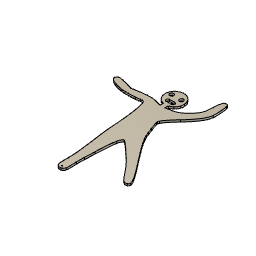
human (Autodesk Fusion 360 design; units mm, degrees)
Autodesk Fusion 360 part; units mm, degrees
sketch "Sketch1" plane through (0, 0, 0) normal (0, 1, 0) x (1, 0, 0)
  spline S0 degree 3 poles (28.5505, 138.7144) (26.7377, 138.2108) (26.0126, 135.8139) (25.6097, 128.7641) knots 0 0 0 0 1 1 1 1
  spline S1 degree 3 poles (25.6097, 128.7641) (25.1062, 119.7605) (24.5019, 117.988) (20.3324, 113.3552) knots 0 0 0 0 1 1 1 1
  spline S2 degree 3 poles (20.3324, 113.3552) (14.6322, 107.0104) (12.2151, 105.7213) (3.1309, 104.1703) knots 0 0 0 0 1 1 1 1
  spline S3 degree 3 poles (3.1309, 104.1703) (-1.1191, 103.4654) (-3.1132, 103.4654) (-5.5101, 104.1905) knots 0 0 0 0 1 1 1 1
  spline S4 degree 3 poles (-5.5101, 104.1905) (-13.4462, 106.6277) (-16.2057, 106.668) (-28.8752, 104.5732) knots 0 0 0 0 1 1 1 1
  line L0 (-28.8752, 104.5732) -> (-33.3267, 103.8481)
  line L1 (-33.3267, 103.8481) -> (-36.8314, 104.8552)
  spline S5 degree 3 poles (-36.8314, 104.8552) (-44.1632, 106.9701) (-47.4061, 107.6348) (-49.1182, 107.3931) knots 0 0 0 0 1 1 1 1
  spline S6 degree 3 poles (-49.1182, 107.3931) (-50.9915, 107.1111) (-51.918, 105.1775) (-50.931, 103.6064) knots 0 0 0 0 1 1 1 1
  spline S7 degree 3 poles (-50.931, 103.6064) (-49.6218, 101.4713) (-43.5388, 99.0945) (-37.2343, 98.2284) knots 0 0 0 0 1 1 1 1
  spline S8 degree 3 poles (-37.2343, 98.2284) (-34.5956, 97.8658) (-26.9818, 97.9262) (-23.4368, 98.3291) knots 0 0 0 0 1 1 1 1
  spline S9 degree 3 poles (-23.4368, 98.3291) (-21.8858, 98.4902) (-19.6702, 98.7521) (-18.5019, 98.8729) knots 0 0 0 0 1 1 1 1
  spline S10 degree 3 poles (-18.5019, 98.8729) (-15.259, 99.2556) (-15.1986, 99.2153) (-14.1915, 96.1336) knots 0 0 0 0 1 1 1 1
  spline S11 degree 3 poles (-14.1915, 96.1336) (-12.3384, 90.4534) (-10.6464, 78.8917) (-9.74, 65.618) knots 0 0 0 0 1 1 1 1
  spline S12 degree 3 poles (-9.74, 65.618) (-9.1358, 56.8762) (-8.3502, 49.6048) (-7.1215, 41.3465) knots 0 0 0 0 1 1 1 1
  spline S13 degree 3 poles (-7.1215, 41.3465) (-6.5173, 37.318) (-5.7518, 31.4365) (-4.4829, 20.902) knots 0 0 0 0 1 1 1 1
  spline S14 degree 3 poles (-4.4829, 20.902) (-4.2613, 19.049) (-4.1002, 15.5039) (-3.9995, 9.8238) knots 0 0 0 0 1 1 1 1
  spline S15 degree 3 poles (-3.9995, 9.8238) (-3.8383, 0.3972) (-3.7779, -0.1265) (-2.4082, -1.4761) knots 0 0 0 0 1 1 1 1
  spline S16 degree 3 poles (-2.4082, -1.4761) (-1.5018, -2.3825) (-0.2933, -2.6443) (1.3584, -2.2818) knots 0 0 0 0 1 1 1 1
  spline S17 degree 3 poles (1.3584, -2.2818) (2.7079, -1.9796) (3.4935, -1.1336) (3.856, 0.377) knots 0 0 0 0 1 1 1 1
  spline S18 degree 3 poles (3.856, 0.377) (4.1582, 1.5856) (4.1783, 5.2515) (3.9567, 10.7302) knots 0 0 0 0 1 1 1 1
  spline S19 degree 3 poles (3.9567, 10.7302) (3.8762, 12.6638) (3.9165, 16.3096) (4.0373, 19.0087) knots 0 0 0 0 1 1 1 1
  spline S20 degree 3 poles (4.0373, 19.0087) (4.1582, 21.6473) (4.3596, 26.2196) (4.4603, 29.1604) knots 0 0 0 0 1 1 1 1
  spline S21 degree 3 poles (4.4603, 29.1604) (4.8631, 38.9093) (5.4674, 46.2008) (6.1925, 49.6451) knots 0 0 0 0 1 1 1 1
  spline S22 degree 3 poles (6.1925, 49.6451) (6.8371, 52.747) (7.8442, 54.5397) (8.952, 54.5397) knots 0 0 0 0 1 1 1 1
  spline S23 degree 3 poles (8.952, 54.5397) (9.7174, 54.5397) (13.9876, 50.8738) (22.4272, 42.9176) knots 0 0 0 0 1 1 1 1
  spline S24 degree 3 poles (22.4272, 42.9176) (30.464, 35.3441) (34.0494, 31.4365) (39.9108, 23.9234) knots 0 0 0 0 1 1 1 1
  spline S25 degree 3 poles (39.9108, 23.9234) (44.8255, 17.5987) (46.6383, 16.37) (49.1158, 17.639) knots 0 0 0 0 1 1 1 1
  spline S26 degree 3 poles (49.1158, 17.639) (50.1833, 18.203) (50.4653, 18.7065) (50.3042, 19.8345) knots 0 0 0 0 1 1 1 1
  spline S27 degree 3 poles (50.3042, 19.8345) (49.9013, 22.7954) (46.3362, 28.113) (34.7745, 43.0586) knots 0 0 0 0 1 1 1 1
  spline S28 degree 3 poles (34.7745, 43.0586) (22.5682, 58.8099) (18.2981, 65.054) (15.8407, 70.6535) knots 0 0 0 0 1 1 1 1
  spline S29 degree 3 poles (15.8407, 70.6535) (13.8265, 75.2863) (10.6641, 83.8065) (9.9793, 86.4854) knots 0 0 0 0 1 1 1 1
  line L2 (9.9793, 86.4854) -> (9.6167, 87.8954)
  line L3 (9.6167, 87.8954) -> (10.2411, 89.2046)
  spline S30 degree 3 poles (10.2411, 89.2046) (11.349, 91.5411) (14.3905, 95.3883) (19.849, 101.2497) knots 0 0 0 0 1 1 1 1
  spline S31 degree 3 poles (19.849, 101.2497) (28.4699, 110.5555) (31.9143, 116.0543) (32.6797, 121.7546) knots 0 0 0 0 1 1 1 1
  spline S32 degree 3 poles (32.6797, 121.7546) (33.0825, 124.8565) (32.5387, 133.1148) (31.6726, 136.4987) knots 0 0 0 0 1 1 1 1
  spline S33 degree 3 poles (31.6726, 136.4987) (31.451, 137.4051) (31.2093, 137.9087) (30.8467, 138.1706) knots 0 0 0 0 1 1 1 1
  spline S34 degree 3 poles (30.8467, 138.1706) (30.1417, 138.6741) (29.2353, 138.8957) (28.5505, 138.7144) knots 0 0 0 0 1 1 1 1
  spline S35 degree 3 poles (-3.9793, 125.924) (-6.5173, 125.2392) (-9.1156, 123.1645) (-10.2234, 120.9287) knots 0 0 0 0 1 1 1 1
  spline S36 degree 3 poles (-10.2234, 120.9287) (-12.8419, 115.591) (-10.2637, 109.2261) (-4.7246, 107.3125) knots 0 0 0 0 1 1 1 1
  spline S37 degree 3 poles (-4.7246, 107.3125) (-1.2803, 106.1241) (2.3856, 106.9097) (5.0243, 109.4073) knots 0 0 0 0 1 1 1 1
  spline S38 degree 3 poles (5.0243, 109.4073) (6.394, 110.6763) (7.1392, 111.8244) (7.7032, 113.4962) knots 0 0 0 0 1 1 1 1
  spline S39 degree 3 poles (7.7032, 113.4962) (8.0658, 114.5839) (8.1262, 115.1479) (8.0456, 116.9406) knots 0 0 0 0 1 1 1 1
  spline S40 degree 3 poles (8.0456, 116.9406) (7.9852, 118.9347) (7.9248, 119.2166) (7.1997, 120.6669) knots 0 0 0 0 1 1 1 1
  spline S41 degree 3 poles (7.1997, 120.6669) (5.1653, 124.8766) (0.4117, 127.1124) (-3.9793, 125.924) knots 0 0 0 0 1 1 1 1
  line L4 (1.3199, 107.2081) -> (1.3199, 103.8951)
  line L5 (-3.5162, 106.9777) -> (-3.5162, 103.7492)
  circle A0 centre (3, 119) radius 2
  circle A1 centre (-7, 119) radius 2
  line L6 (-4, 110.2788) -> (1.4991, 110.2788)
  arc A2 (1.4991, 110.2788) -> (1.4991, 113.7212) centre (1.4991, 112) ccw
  line L7 (1.4991, 113.7212) -> (-4, 113.7212)
  arc A3 (-4, 113.7212) -> (-4, 110.2788) centre (-4, 112) ccw
  line L8 (-4, 112) -> (1.4991, 112) construction
  dimension "d1" = 4
  dimension "d2" = 4
  constraint coincident S37 L4.start
  constraint coincident S3 L4.end
  constraint vertical L4
  constraint coincident S37 L5.start
  constraint coincident S3 L5.end
  constraint parallel L4 L5
  constraint tangent L6 A2
  constraint tangent A2 L7
  constraint parallel L6 L7
  constraint tangent L7 A3
  constraint tangent L6 A3
  constraint horizontal L8
  measures "d1" diameter of A0
  measures "d2" diameter of A1
extrude "Extrude1" add sketch "Sketch1" along normal blind 2
sketch "Sketch2" plane through (0, 2, 0) normal (0, 1, 0) x (-1, 0, 0)
  arc A0 (4, -113.7212) -> (4, -110.2788) centre (4, -112) ccw
  line L0 (4, -113.7212) -> (-1.4991, -113.7212)
  arc A1 (-1.4991, -110.2788) -> (-1.4991, -113.7212) centre (-1.4991, -112) ccw
  line L1 (-1.4991, -110.2788) -> (4, -110.2788)
  circle A2 centre (-3, -119) radius 2
  circle A3 centre (7, -119) radius 2
  spline S0 degree 3 poles (-1.3199, -107.2081) (-2.6712, -107.6373) (-3.9352, -108.3765) (-5.0243, -109.4073) knots 0.587264 0.587264 0.587264 0.587264 1 1 1 1
  spline S1 degree 3 poles (-5.0243, -109.4073) (-6.394, -110.6763) (-7.1392, -111.8244) (-7.7032, -113.4962) knots 0 0 0 0 1 1 1 1
  spline S2 degree 3 poles (-7.7032, -113.4962) (-8.0658, -114.5839) (-8.1262, -115.1479) (-8.0456, -116.9406) knots 0 0 0 0 1 1 1 1
  spline S3 degree 3 poles (-8.0456, -116.9406) (-7.9852, -118.9347) (-7.9248, -119.2166) (-7.1997, -120.6669) knots 0 0 0 0 1 1 1 1
  spline S4 degree 3 poles (-7.1997, -120.6669) (-5.1653, -124.8766) (-0.4117, -127.1124) (3.9793, -125.924) knots 0 0 0 0 1 1 1 1
  spline S5 degree 3 poles (3.9793, -125.924) (6.5173, -125.2392) (9.1156, -123.1645) (10.2234, -120.9287) knots 0 0 0 0 1 1 1 1
  spline S6 degree 3 poles (10.2234, -120.9287) (12.8419, -115.591) (10.2637, -109.2261) (4.7246, -107.3125) knots 0 0 0 0 1 1 1 1
  spline S7 degree 3 poles (4.7246, -107.3125) (4.3241, -107.1744) (3.9207, -107.0629) (3.5162, -106.9777) knots 0 0 0 0 0.116263 0.116263 0.116263 0.116263
  line L2 (3.5162, -106.9777) -> (3.5162, -103.7492)
  spline S8 degree 3 poles (3.5162, -103.7492) (4.1886, -103.8388) (4.8333, -103.9857) (5.5101, -104.1905) knots 0.717636 0.717636 0.717636 0.717636 1 1 1 1
  spline S9 degree 3 poles (5.5101, -104.1905) (13.4462, -106.6277) (16.2057, -106.668) (28.8752, -104.5732) knots 0 0 0 0 1 1 1 1
  line L3 (28.8752, -104.5732) -> (33.3267, -103.8481)
  line L4 (33.3267, -103.8481) -> (36.8314, -104.8552)
  spline S10 degree 3 poles (36.8314, -104.8552) (44.1632, -106.9701) (47.4061, -107.6348) (49.1182, -107.3931) knots 0 0 0 0 1 1 1 1
  spline S11 degree 3 poles (49.1182, -107.3931) (50.9915, -107.1111) (51.918, -105.1775) (50.931, -103.6064) knots 0 0 0 0 1 1 1 1
  spline S12 degree 3 poles (50.931, -103.6064) (49.6218, -101.4713) (43.5388, -99.0945) (37.2343, -98.2284) knots 0 0 0 0 1 1 1 1
  spline S13 degree 3 poles (37.2343, -98.2284) (34.5956, -97.8658) (26.9818, -97.9262) (23.4368, -98.3291) knots 0 0 0 0 1 1 1 1
  spline S14 degree 3 poles (23.4368, -98.3291) (21.8858, -98.4902) (19.6702, -98.7521) (18.5019, -98.8729) knots 0 0 0 0 1 1 1 1
  spline S15 degree 3 poles (18.5019, -98.8729) (15.259, -99.2556) (15.1986, -99.2153) (14.1915, -96.1336) knots 0 0 0 0 1 1 1 1
  spline S16 degree 3 poles (14.1915, -96.1336) (12.3384, -90.4534) (10.6464, -78.8917) (9.74, -65.618) knots 0 0 0 0 1 1 1 1
  spline S17 degree 3 poles (9.74, -65.618) (9.1358, -56.8762) (8.3502, -49.6048) (7.1215, -41.3465) knots 0 0 0 0 1 1 1 1
  spline S18 degree 3 poles (7.1215, -41.3465) (6.5173, -37.318) (5.7518, -31.4365) (4.4829, -20.902) knots 0 0 0 0 1 1 1 1
  spline S19 degree 3 poles (4.4829, -20.902) (4.2613, -19.049) (4.1002, -15.5039) (3.9995, -9.8238) knots 0 0 0 0 1 1 1 1
  spline S20 degree 3 poles (3.9995, -9.8238) (3.8383, -0.3972) (3.7779, 0.1265) (2.4082, 1.4761) knots 0 0 0 0 1 1 1 1
  spline S21 degree 3 poles (2.4082, 1.4761) (1.5018, 2.3825) (0.2933, 2.6443) (-1.3584, 2.2818) knots 0 0 0 0 1 1 1 1
  spline S22 degree 3 poles (-1.3584, 2.2818) (-2.7079, 1.9796) (-3.4935, 1.1336) (-3.856, -0.377) knots 0 0 0 0 1 1 1 1
  spline S23 degree 3 poles (-3.856, -0.377) (-4.1582, -1.5856) (-4.1783, -5.2515) (-3.9567, -10.7302) knots 0 0 0 0 1 1 1 1
  spline S24 degree 3 poles (-3.9567, -10.7302) (-3.8762, -12.6638) (-3.9165, -16.3096) (-4.0373, -19.0087) knots 0 0 0 0 1 1 1 1
  spline S25 degree 3 poles (-4.0373, -19.0087) (-4.1582, -21.6473) (-4.3596, -26.2196) (-4.4603, -29.1604) knots 0 0 0 0 1 1 1 1
  spline S26 degree 3 poles (-4.4603, -29.1604) (-4.8631, -38.9093) (-5.4674, -46.2008) (-6.1925, -49.6451) knots 0 0 0 0 1 1 1 1
  spline S27 degree 3 poles (-6.1925, -49.6451) (-6.8371, -52.747) (-7.8442, -54.5397) (-8.952, -54.5397) knots 0 0 0 0 1 1 1 1
  spline S28 degree 3 poles (-8.952, -54.5397) (-9.7174, -54.5397) (-13.9876, -50.8738) (-22.4272, -42.9176) knots 0 0 0 0 1 1 1 1
  spline S29 degree 3 poles (-22.4272, -42.9176) (-30.464, -35.3441) (-34.0494, -31.4365) (-39.9108, -23.9234) knots 0 0 0 0 1 1 1 1
  spline S30 degree 3 poles (-39.9108, -23.9234) (-44.8255, -17.5987) (-46.6383, -16.37) (-49.1158, -17.639) knots 0 0 0 0 1 1 1 1
  spline S31 degree 3 poles (-49.1158, -17.639) (-50.1833, -18.203) (-50.4653, -18.7065) (-50.3042, -19.8345) knots 0 0 0 0 1 1 1 1
  spline S32 degree 3 poles (-50.3042, -19.8345) (-49.9013, -22.7954) (-46.3362, -28.113) (-34.7745, -43.0586) knots 0 0 0 0 1 1 1 1
  spline S33 degree 3 poles (-34.7745, -43.0586) (-22.5682, -58.8099) (-18.2981, -65.054) (-15.8407, -70.6535) knots 0 0 0 0 1 1 1 1
  spline S34 degree 3 poles (-15.8407, -70.6535) (-13.8265, -75.2863) (-10.6641, -83.8065) (-9.9793, -86.4854) knots 0 0 0 0 1 1 1 1
  line L5 (-9.9793, -86.4854) -> (-9.6167, -87.8954)
  line L6 (-9.6167, -87.8954) -> (-10.2411, -89.2046)
  spline S35 degree 3 poles (-10.2411, -89.2046) (-11.349, -91.5411) (-14.3905, -95.3883) (-19.849, -101.2497) knots 0 0 0 0 1 1 1 1
  spline S36 degree 3 poles (-19.849, -101.2497) (-28.4699, -110.5555) (-31.9143, -116.0543) (-32.6797, -121.7546) knots 0 0 0 0 1 1 1 1
  spline S37 degree 3 poles (-32.6797, -121.7546) (-33.0825, -124.8565) (-32.5387, -133.1148) (-31.6726, -136.4987) knots 0 0 0 0 1 1 1 1
  spline S38 degree 3 poles (-31.6726, -136.4987) (-31.451, -137.4051) (-31.2093, -137.9087) (-30.8467, -138.1706) knots 0 0 0 0 1 1 1 1
  spline S39 degree 3 poles (-30.8467, -138.1706) (-30.1417, -138.6741) (-29.2353, -138.8957) (-28.5505, -138.7144) knots 0 0 0 0 1 1 1 1
  spline S40 degree 3 poles (-28.5505, -138.7144) (-26.7377, -138.2108) (-26.0126, -135.8139) (-25.6097, -128.7641) knots 0 0 0 0 1 1 1 1
  spline S41 degree 3 poles (-25.6097, -128.7641) (-25.1062, -119.7605) (-24.5019, -117.988) (-20.3324, -113.3552) knots 0 0 0 0 1 1 1 1
  spline S42 degree 3 poles (-20.3324, -113.3552) (-14.6322, -107.0104) (-12.2151, -105.7213) (-3.1309, -104.1703) knots 0 0 0 0 1 1 1 1
  spline S43 degree 3 poles (-3.1309, -104.1703) (-2.4771, -104.0619) (-1.8767, -103.9701) (-1.3199, -103.8951) knots 0 0 0 0 0.15384 0.15384 0.15384 0.15384
  line L7 (-1.3199, -103.8951) -> (-1.3199, -107.2081)
  circle A4 centre (0, 0) radius 0.5
  dimension "d5" = 1
  constraint coincident A4.centre origin
  measures "d5" diameter of A4
extrude "Extrude2" cut sketch "Sketch2" against normal up to surface (2 mm away) contours A4
